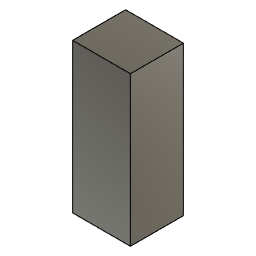
柱設置用太い方［流用可能］※局面はなるべく作るな！ (Autodesk Fusion 360 design; units mm, degrees)
Autodesk Fusion 360 part; units mm, degrees
sketch "スケッチ1" plane through (0, 0, 0) normal (0, 1, 0) x (1, 0, 0)
sketch "スケッチ2" plane through (0, 0, 0) normal (0, 0, 1) x (1, 0, 0)
  line L0 (0, 0) -> (-10000, 0)
  line L1 (-10000, 0) -> (-10000, 8100)
  line L2 (-10000, 8100) -> (0, 8100)
  line L3 (0, 8100) -> (0, 0)
  line L4 (10, -10) -> (-10010, -10)
  line L5 (-10010, -10) -> (-10010, 8110)
  line L6 (-10010, 8110) -> (10, 8110)
  line L7 (10, 8110) -> (10, -10)
  point P0 (10, -10)
  dimension "d1" = 10000
  dimension "d2" = 8100
  dimension "d4" = 10020
  dimension "d5" = 8120
  constraint horizontal L0
  constraint vertical L1
  constraint horizontal L2
  constraint vertical L3
  constraint coincident L0.start L3.end
  constraint horizontal L4
  constraint vertical L5
  constraint horizontal L6
  constraint vertical L7
  constraint coincident P0 L4.start
  measures "d1" distance of L0.start L0.end
  measures "d2" distance of L0.start L2.end
  measures "d4" distance of L5.end L6.end
  measures "d5" distance of L4.end L5.end
sketch "スケッチ3" plane through (0, 0, 0) normal (0, 0, 1) x (1, 0, 0)
sketch "スケッチ4" plane through (0, 0, 0) normal (0, 0, 1) x (1, 0, 0)
  line L0 (0, 0) -> (1200, 0)
  line L1 (1200, 0) -> (1200, 1000)
  line L2 (1200, 1000) -> (0, 1000)
  line L3 (0, 1000) -> (0, 0)
  dimension "d10" = 1200
  dimension "d11" = 1000
  constraint horizontal L0
  constraint vertical L1
  constraint horizontal L2
  constraint vertical L3
  constraint coincident L0.start L3.end
  measures "d10" distance of L1.end L2.end
  measures "d11" distance of L0.end L1.end
extrude "押し出し2" add sketch "スケッチ4" along normal blind 3100
sketch "スケッチ5" plane through (0, 0, 3100) normal (0, 0, 1) x (-1, 0, 0)
  line L0 (0, -1000) -> (0, 0)
  line L1 (0, 0) -> (-1200, 0)
  line L2 (-1200, 0) -> (-1200, -1000)
  line L3 (-1200, -1000) -> (0, -1000)
  line L4 (0, 0) -> (-1200, 0)
  line L5 (-1200, 0) -> (-1200, -100)
  line L6 (-1200, -100) -> (0, -100)
  line L7 (0, -100) -> (0, 0)
  constraint horizontal L4
  constraint vertical L5
  constraint horizontal L6
  constraint vertical L7
  constraint coincident L0.end L1.start
extrude "押し出し3" cut sketch "スケッチ5" against normal blind 3100 contours L0 L1 L2 L4 L5 L6 L7
sketch "スケッチ6" plane through (0, 0, 3100) normal (0, 0, 1) x (-1, 0, 0)
  line L0 (0, -100) -> (-1200, -100)
  line L1 (-1200, -100) -> (-1200, -1000)
  line L2 (-1200, -1000) -> (0, -1000)
  line L3 (0, -1000) -> (0, -100)
  line L4 (0, -1000) -> (-1200, -1000)
  line L5 (-1200, -1000) -> (-1200, -1200)
  line L6 (-1200, -1200) -> (0, -1200)
  line L7 (0, -1200) -> (0, -1000)
  constraint horizontal L4
  constraint vertical L5
  constraint horizontal L6
  constraint vertical L7
  constraint coincident L2.end L3.start
extrude "押し出し4" add sketch "スケッチ6" against normal blind 3100 contours L2 L4 L5 L6 L7
